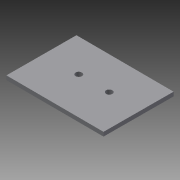
# Autodesk Inventor part: GehäuseBack
Saved by Autodesk Inventor 2014 (Build 180170000, 170)
## iProperties
Created: 2013-05-31
Part Number: GehäuseBack
Material: Generisch
Document SubType Name: Modeling
Designer: hanse
Density: 1 g/cm^3
Appearance: Vorgabe
Author: hanse
Autodesk Inventor part; units mm, degrees
ref_plane "YZ Plane" through (0, 0, 0) normal (1, 0, 0) x (0, 1, 0)
ref_plane "XZ Plane" through (0, 0, 0) normal (0, 1, 0) x (-1, 0, 0)
ref_plane "XY Plane" through (0, 0, 0) normal (0, 0, 1) x (1, 0, 0)
sketch "Skizze1" plane through (0, 0, 0) normal (0, 0, 1) x (1, 0, 0)
  circle A0 centre (-1.772, 1.6716) radius 1.5 projected
  circle A1 centre (-16.7719, 1.7262) radius 1.5 projected
  circle A2 centre (-16.7719, 1.7262) radius 1.55
  circle A3 centre (-1.772, 1.6716) radius 1.55
  arc A4 (6.6108, 4.9468) -> (6.4575, -1.9719) centre (-1.772, 1.6716) ccw projected
  line L0 (6.6108, 4.9468) -> (13.7945, 4.9207) projected
  line L1 (13.7693, -1.9985) -> (6.4575, -1.9719) projected
  circle A5 centre (-16.7719, 1.7262) radius 1.45 projected
  line L2 (13.7161, -16.6303) -> (-34.0833, -16.4565) projected
  line L3 (13.8407, 17.6149) -> (13.7945, 4.9207) projected
  line L4 (-33.9587, 17.7888) -> (13.8407, 17.6149) projected
  line L5 (-34.0833, -16.4565) -> (-33.9587, 17.7888) projected
  line L6 (13.7693, -1.9985) -> (13.7161, -16.6303) projected
  line L7 (13.7693, -1.9985) -> (13.7945, 4.9207)
  point P0 (0, 0)
  dimension "d0" = 3.1
  dimension "d1" = 3.1
  constraints: 2 centre point, 2 coincident, 2 end point, 1 collinear
  measures "d0" diameter of A2
  measures "d1" diameter of A3
extrude "Extrusion1" add sketch "Skizze1" along normal blind 2 contours L0 L7 L1 A4 | A4 L1 L6 L2 L5 L4 L3 L0
sketch "Skizze2" plane through (0, 0, 0) normal (0, 0, -1) x (-1, 0, 0)
  circle A0 centre (1.772, 1.6716) radius 1.55 projected
  circle A1 centre (1.772, 1.6716) radius 3.55
  point P0 (0, 0)
  dimension "d13" = 2
  constraints: 1 centre point, 1 coincident
  measures "d13" radial gap between concentric circles of A0 A1
extrude "Extrusion2" add sketch "Skizze2" along normal blind 3.5
fillet "Rundung1" radius 2 1 edges at (1.778, 1.6716, 0)
